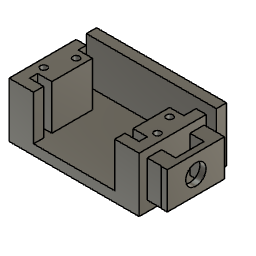
hub right down v4 (Autodesk Fusion 360 design; units mm, degrees)
Autodesk Fusion 360 part; units mm, degrees
sketch "Sketch1" plane through (0, 0, 0) normal (0, 0, 1) x (1, 0, 0) in component "casing v1"
  line L0 (-13.5, -7.7959) -> (9.5, -7.7959)
  line L1 (9.5, -7.7959) -> (9.5, -4.7959)
  line L2 (9.5, -4.7959) -> (19.5, -4.7959)
  line L3 (19.5, -4.7959) -> (19.5, 1.2041)
  line L4 (19.5, 1.2041) -> (26.5, 1.2041)
  line L5 (26.5, 1.2041) -> (26.5, 4.2041)
  line L6 (26.5, 4.2041) -> (19.5, 4.2041)
  line L7 (19.5, 4.2041) -> (19.5, 30.2041)
  line L8 (19.5, 30.2041) -> (-19.5, 30.2041)
  line L9 (-19.5, 30.2041) -> (-19.5, 4.2041)
  line L10 (-19.5, 4.2041) -> (-26.5, 4.2041)
  line L11 (-26.5, 4.2041) -> (-26.5, 1.2041)
  line L12 (-26.5, 1.2041) -> (-19.5, 1.2041)
  line L13 (-19.5, 1.2041) -> (-19.5, -4.7959)
  line L14 (-19.5, -4.7959) -> (-13.5, -4.7959)
  line L15 (-13.5, -4.7959) -> (-13.5, -7.7959)
  line L16 (-20, 0.7041) -> (-32, 0.7041)
  line L17 (-32, 0.7041) -> (-32, -4.2959)
  line L18 (-32, -4.2959) -> (-20, -4.2959)
  line L19 (-20, -4.2959) -> (-20, 0.7041)
  line L20 (-32, 0.7041) -> (-27, 0.7041)
  line L21 (-27, 0.7041) -> (-27, 38.7041)
  line L22 (-27, 38.7041) -> (-32, 38.7041)
  line L23 (-32, 38.7041) -> (-32, 0.7041)
  line L24 (-27, 38.7041) -> (27, 38.7041)
  line L25 (27, 38.7041) -> (27, 33.7041)
  line L26 (27, 33.7041) -> (-27, 33.7041)
  line L27 (-27, 33.7041) -> (-27, 38.7041)
  line L28 (20, 0.7041) -> (32, 0.7041)
  line L29 (32, 0.7041) -> (32, -4.2959)
  line L30 (32, -4.2959) -> (20, -4.2959)
  line L31 (20, -4.2959) -> (20, 0.7041)
  line L32 (32, 0.7041) -> (27, 0.7041)
  line L33 (27, 0.7041) -> (27, 38.7041)
  line L34 (27, 38.7041) -> (32, 38.7041)
  line L35 (32, 38.7041) -> (32, 0.7041)
  line L36 (27, 4.7041) -> (20, 4.7041)
  line L37 (20, 4.7041) -> (20, 22.7041)
  line L38 (20, 22.7041) -> (27, 22.7041)
  line L39 (27, 22.7041) -> (27, 4.7041)
  line L40 (-27, 4.7041) -> (-20, 4.7041)
  line L41 (-20, 4.7041) -> (-20, 24.7041)
  line L42 (-20, 24.7041) -> (-27, 24.7041)
  line L43 (-27, 24.7041) -> (-27, 4.7041)
  line L44 (-32, 38.7041) -> (32, 38.7041)
  line L45 (32, 38.7041) -> (32, -4.2959)
  line L46 (32, -4.2959) -> (-32, -4.2959)
  line L47 (-32, -4.2959) -> (-32, 38.7041)
  line L48 (-27, 33.7041) -> (-32, 33.7041)
  line L49 (-32, 33.7041) -> (-32, 28.7041)
  line L50 (-32, 28.7041) -> (-27, 28.7041)
  line L51 (-27, 28.7041) -> (-27, 33.7041)
  line L52 (27, 33.7041) -> (32, 33.7041)
  line L53 (32, 33.7041) -> (32, 28.7041)
  line L54 (32, 28.7041) -> (27, 28.7041)
  line L55 (27, 28.7041) -> (27, 33.7041)
  dimension "d34" = 0.5
  dimension "d35" = 0.5
  dimension "d36" = 5
  dimension "d37" = 12
  dimension "d38" = 0.5
  dimension "d39" = 3.5
  dimension "d40" = 5
  dimension "d41" = 0.5
  dimension "d42" = 0.5
  dimension "d43" = 12
  dimension "d44" = 5
  dimension "d45" = 0.5
  dimension "d46" = 0.5
  dimension "d47" = 0.5
  dimension "d48" = 18
  dimension "d49" = 0.5
  dimension "d50" = 0.5
  dimension "d51" = 20
  dimension "d56" = 5
  dimension "d57" = 5
  constraint horizontal L16
  constraint vertical L17
  constraint horizontal L18
  constraint vertical L19
  constraint horizontal L20
  constraint vertical L21
  constraint horizontal L22
  constraint vertical L23
  constraint horizontal L24
  constraint vertical L25
  constraint horizontal L26
  constraint vertical L27
  constraint horizontal L28
  constraint vertical L29
  constraint horizontal L30
  constraint vertical L31
  constraint horizontal L32
  constraint vertical L33
  constraint horizontal L34
  constraint vertical L35
  constraint horizontal L36
  constraint vertical L37
  constraint horizontal L38
  constraint vertical L39
  constraint coincident L33 L36.start
  constraint horizontal L40
  constraint vertical L41
  constraint horizontal L42
  constraint vertical L43
  constraint coincident L21 L40.start
  constraint horizontal L44
  constraint vertical L45
  constraint horizontal L46
  constraint vertical L47
  constraint horizontal L48
  constraint vertical L49
  constraint horizontal L50
  constraint vertical L51
  constraint coincident L47 L49.end
  constraint horizontal L52
  constraint vertical L53
  constraint horizontal L54
  constraint vertical L55
  constraint coincident L45 L53.end
  measures "d34" distance of L13 L19
  measures "d35" distance of L12 L16
  measures "d36" distance of L16.end L17.end
  measures "d37" distance of L17.end L18.end
  measures "d38" distance of L11 L21
  measures "d39" distance of L8 L26
  measures "d40" distance of L24.end L25.end
  measures "d41" distance of L4 L28
  measures "d42" distance of L3 L31
  measures "d43" distance of L29.end L30.end
  measures "d44" distance of L28.end L29.end
  measures "d45" distance of L5 L33
  measures "d46" distance of L6 L36
  measures "d47" distance of L7 L37
  measures "d48" distance of L36.end L37.end
  measures "d49" distance of L10 L40
  measures "d50" distance of L9 L41
  measures "d51" distance of L40 L42
  measures "d56" distance of L48 L50
  measures "d57" distance of L52 L54
extrude "Extrude1" add sketch "Sketch1" against normal blind 5 contours L3 L4 L5 L6 L7 L8 L9 L10 L11 L12 L13 L16 L19 L21 L26 L28 L31 L33 L36 L37 L38 L40 L41 L42 L46 L51 L55 | L3 L4 L5 L6 L7 L8 L9 L10 L11 L12 L13 L46 | L16 L17 L18 L19 L20 L46 L47 | L28 L29 L30 L31 L32 L45 L46 | L16 L20 L21 L23 L43 L47 L50 | L28 L32 L33 L35 L39 L45 L54 | L21 L23 L47 L48 L49 L50 L51 | L21 L40 L41 L42 L43 | L33 L35 L45 L52 L53 L54 L55 | L33 L36 L37 L38 L39 | L21 L22 L23 L27 L44 L47 L48 | L25 L33 L34 L35 L44 L45 L52 | L21 L24 L25 L26 L27 L33 L44 makes body 1 in component "casing v1"
extrude "Extrude2" add sketch "Sketch1" along normal blind 22 contours L16 L17 L18 L19 L20 L46 L47 | L28 L29 L30 L31 L32 L45 L46 | L16 L20 L21 L23 L43 L47 L50 | L28 L32 L33 L35 L39 L45 L54 | L21 L40 L41 L42 L43 | L33 L36 L37 L38 L39 | L21 L22 L23 L27 L44 L47 L48 | L25 L33 L34 L35 L44 L45 L52 | L21 L24 L25 L26 L27 L33 L44 bodies 1 in component "casing v1"
sketch "Sketch1 (2)" plane through (0, 0, 22) normal (0, 0, 1) x (-1, 0, 0)
  line L0 (20, 4.2959) -> (20, -0.7041)
  line L1 (20, -0.7041) -> (27, -0.7041)
  line L2 (27, -0.7041) -> (27, -4.7041)
  line L3 (27, -4.7041) -> (20, -4.7041)
  line L4 (20, -4.7041) -> (20, -24.7041)
  line L5 (20, -24.7041) -> (27, -24.7041)
  line L6 (27, -24.7041) -> (27, -28.7041)
  line L7 (27, -28.7041) -> (32, -28.7041)
  line L8 (32, -28.7041) -> (32, 4.2959)
  line L9 (32, 4.2959) -> (20, 4.2959)
  line L10 (-32, 4.2959) -> (-32, -28.7041)
  line L11 (-32, -28.7041) -> (-27, -28.7041)
  line L12 (-27, -28.7041) -> (-27, -22.7041)
  line L13 (-27, -22.7041) -> (-20, -22.7041)
  line L14 (-20, -22.7041) -> (-20, -4.7041)
  line L15 (-20, -4.7041) -> (-27, -4.7041)
  line L16 (-27, -4.7041) -> (-27, -0.7041)
  line L17 (-27, -0.7041) -> (-20, -0.7041)
  line L18 (-20, -0.7041) -> (-20, 4.2959)
  line L19 (-20, 4.2959) -> (-32, 4.2959)
  circle A0 centre (24, -20.7041) radius 1.65
  circle A1 centre (28, -8.7041) radius 1.65
  circle A2 centre (-24, -18.7041) radius 1.65
  circle A3 centre (-28, -8.7041) radius 1.65
  dimension "d1" = 3.3
  dimension "d2" = 3.3
  dimension "d3" = 3.3
  dimension "d4" = 3.3
  dimension "d5" = 4
  dimension "d6" = 4
  dimension "d7" = 4
  dimension "d8" = 4
  dimension "d9" = 4
  dimension "d10" = 4
  dimension "d11" = 4
  dimension "d12" = 4
  measures "d1" diameter of A0
  measures "d2" diameter of A1
  measures "d3" diameter of A2
  measures "d4" diameter of A3
  measures "d5" distance of L4 A0.centre
  measures "d6" distance of L5 A0.centre
  measures "d7" distance of L8 A1.centre
  measures "d8" distance of L3 A1.centre
  measures "d9" distance of L13 A2.centre
  measures "d10" distance of L14 A2.centre
  measures "d11" distance of L15 A3.centre
  measures "d12" distance of L10 A3.centre
extrude "Extrude3" cut sketch "Sketch1 (2)" against normal blind 5 contours A0 | A1 | A2 | A3 bodies 1 in component "casing v1"
sketch "Sketch1 (3)" plane through (0, 0, 0) normal (0, 0, 1) x (1, 0, 0) in component "casing v1 (1)"
  line L0 (-13.5, -7.7959) -> (9.5, -7.7959)
  line L1 (9.5, -7.7959) -> (9.5, -4.7959)
  line L2 (9.5, -4.7959) -> (19.5, -4.7959)
  line L3 (19.5, -4.7959) -> (19.5, 1.2041)
  line L4 (19.5, 1.2041) -> (26.5, 1.2041)
  line L5 (26.5, 1.2041) -> (26.5, 4.2041)
  line L6 (26.5, 4.2041) -> (19.5, 4.2041)
  line L7 (19.5, 4.2041) -> (19.5, 30.2041)
  line L8 (19.5, 30.2041) -> (-19.5, 30.2041)
  line L9 (-19.5, 30.2041) -> (-19.5, 4.2041)
  line L10 (-19.5, 4.2041) -> (-26.5, 4.2041)
  line L11 (-26.5, 4.2041) -> (-26.5, 1.2041)
  line L12 (-26.5, 1.2041) -> (-19.5, 1.2041)
  line L13 (-19.5, 1.2041) -> (-19.5, -4.7959)
  line L14 (-19.5, -4.7959) -> (-13.5, -4.7959)
  line L15 (-13.5, -4.7959) -> (-13.5, -7.7959)
  line L16 (-20, 0.7041) -> (-32, 0.7041)
  line L17 (-32, 0.7041) -> (-32, -4.2959)
  line L18 (-32, -4.2959) -> (-20, -4.2959)
  line L19 (-20, -4.2959) -> (-20, 0.7041)
  line L20 (-32, 0.7041) -> (-27, 0.7041)
  line L21 (-27, 0.7041) -> (-27, 38.7041)
  line L22 (-27, 38.7041) -> (-32, 38.7041)
  line L23 (-32, 38.7041) -> (-32, 0.7041)
  line L24 (-27, 38.7041) -> (27, 38.7041)
  line L25 (27, 38.7041) -> (27, 33.7041)
  line L26 (27, 33.7041) -> (-27, 33.7041)
  line L27 (-27, 33.7041) -> (-27, 38.7041)
  line L28 (20, 0.7041) -> (32, 0.7041)
  line L29 (32, 0.7041) -> (32, -4.2959)
  line L30 (32, -4.2959) -> (20, -4.2959)
  line L31 (20, -4.2959) -> (20, 0.7041)
  line L32 (32, 0.7041) -> (27, 0.7041)
  line L33 (27, 0.7041) -> (27, 38.7041)
  line L34 (27, 38.7041) -> (32, 38.7041)
  line L35 (32, 38.7041) -> (32, 0.7041)
  line L36 (27, 4.7041) -> (20, 4.7041)
  line L37 (20, 4.7041) -> (20, 22.7041)
  line L38 (20, 22.7041) -> (27, 22.7041)
  line L39 (27, 22.7041) -> (27, 4.7041)
  line L40 (-27, 4.7041) -> (-20, 4.7041)
  line L41 (-20, 4.7041) -> (-20, 24.7041)
  line L42 (-20, 24.7041) -> (-27, 24.7041)
  line L43 (-27, 24.7041) -> (-27, 4.7041)
  line L44 (-32, 38.7041) -> (32, 38.7041)
  line L45 (32, 38.7041) -> (32, -4.2959)
  line L46 (32, -4.2959) -> (-32, -4.2959)
  line L47 (-32, -4.2959) -> (-32, 38.7041)
  line L48 (-27, 33.7041) -> (-32, 33.7041)
  line L49 (-32, 33.7041) -> (-32, 28.7041)
  line L50 (-32, 28.7041) -> (-27, 28.7041)
  line L51 (-27, 28.7041) -> (-27, 33.7041)
  line L52 (27, 33.7041) -> (32, 33.7041)
  line L53 (32, 33.7041) -> (32, 28.7041)
  line L54 (32, 28.7041) -> (27, 28.7041)
  line L55 (27, 28.7041) -> (27, 33.7041)
  dimension "d34_1" = 0.5
  dimension "d35_1" = 0.5
  dimension "d36_1" = 5
  dimension "d37_1" = 12
  dimension "d38_1" = 0.5
  dimension "d39_1" = 3.5
  dimension "d40_1" = 5
  dimension "d41_1" = 0.5
  dimension "d42_1" = 0.5
  dimension "d43_1" = 12
  dimension "d44_1" = 5
  dimension "d45_1" = 0.5
  dimension "d46_1" = 0.5
  dimension "d47_1" = 0.5
  dimension "d48_1" = 18
  dimension "d49_1" = 0.5
  dimension "d50_1" = 0.5
  dimension "d51_1" = 20
  dimension "d56_1" = 5
  dimension "d57_1" = 5
  constraint horizontal L16
  constraint vertical L17
  constraint horizontal L18
  constraint vertical L19
  constraint horizontal L20
  constraint vertical L21
  constraint horizontal L22
  constraint vertical L23
  constraint horizontal L24
  constraint vertical L25
  constraint horizontal L26
  constraint vertical L27
  constraint horizontal L28
  constraint vertical L29
  constraint horizontal L30
  constraint vertical L31
  constraint horizontal L32
  constraint vertical L33
  constraint horizontal L34
  constraint vertical L35
  constraint horizontal L36
  constraint vertical L37
  constraint horizontal L38
  constraint vertical L39
  constraint coincident L33 L36.start
  constraint horizontal L40
  constraint vertical L41
  constraint horizontal L42
  constraint vertical L43
  constraint coincident L21 L40.start
  constraint horizontal L44
  constraint vertical L45
  constraint horizontal L46
  constraint vertical L47
  constraint horizontal L48
  constraint vertical L49
  constraint horizontal L50
  constraint vertical L51
  constraint coincident L47 L49.end
  constraint horizontal L52
  constraint vertical L53
  constraint horizontal L54
  constraint vertical L55
  constraint coincident L45 L53.end
  measures "d34_1" distance of L13 L19
  measures "d35_1" distance of L12 L16
  measures "d36_1" distance of L16.end L17.end
  measures "d37_1" distance of L17.end L18.end
  measures "d38_1" distance of L11 L21
  measures "d39_1" distance of L8 L26
  measures "d40_1" distance of L24.end L25.end
  measures "d41_1" distance of L4 L28
  measures "d42_1" distance of L3 L31
  measures "d43_1" distance of L29.end L30.end
  measures "d44_1" distance of L28.end L29.end
  measures "d45_1" distance of L5 L33
  measures "d46_1" distance of L6 L36
  measures "d47_1" distance of L7 L37
  measures "d48_1" distance of L36.end L37.end
  measures "d49_1" distance of L10 L40
  measures "d50_1" distance of L9 L41
  measures "d51_1" distance of L40 L42
  measures "d56_1" distance of L48 L50
  measures "d57_1" distance of L52 L54
extrude "Extrude1'" add sketch "Sketch1 (3)" against normal blind 5 separate body contours L3 L4 L5 L6 L7 L8 L9 L10 L11 L12 L13 L16 L19 L21 L26 L28 L31 L33 L36 L37 L38 L40 L41 L42 L46 L51 L55 | L3 L4 L5 L6 L7 L8 L9 L10 L11 L12 L13 L46 | L16 L17 L18 L19 L20 L46 L47 | L28 L29 L30 L31 L32 L45 L46 | L16 L20 L21 L23 L43 L47 L50 | L28 L32 L33 L35 L39 L45 L54 | L21 L23 L47 L48 L49 L50 L51 | L21 L40 L41 L42 L43 | L33 L35 L45 L52 L53 L54 L55 | L33 L36 L37 L38 L39 | L21 L22 L23 L27 L44 L47 L48 | L25 L33 L34 L35 L44 L45 L52 | L21 L24 L25 L26 L27 L33 L44 makes body 2 in component "casing v1 (1)"
extrude "Extrude2'" add sketch "Sketch1 (3)" along normal blind 22 contours L16 L17 L18 L19 L20 L46 L47 | L28 L29 L30 L31 L32 L45 L46 | L16 L20 L21 L23 L43 L47 L50 | L28 L32 L33 L35 L39 L45 L54 | L21 L40 L41 L42 L43 | L33 L36 L37 L38 L39 | L21 L22 L23 L27 L44 L47 L48 | L25 L33 L34 L35 L44 L45 L52 | L21 L24 L25 L26 L27 L33 L44 bodies 2 in component "casing v1 (1)"
sketch "Sketch2" plane through (0, 0, 41.3886) normal (0, 0, -1) x (1, 0, 0)
  line L0 (-31.9538, 4.2959) -> (-31.9538, -28.7041)
  line L1 (-31.9538, -28.7041) -> (-26.9538, -28.7041)
  line L2 (-26.9538, -28.7041) -> (-26.9538, -22.7041)
  line L3 (-26.9538, -22.7041) -> (-19.9538, -22.7041)
  line L4 (-19.9538, -22.7041) -> (-19.9538, -4.7041)
  line L5 (-19.9538, -4.7041) -> (-26.9538, -4.7041)
  line L6 (-26.9538, -4.7041) -> (-26.9538, -0.7041)
  line L7 (-26.9538, -0.7041) -> (-19.9538, -0.7041)
  line L8 (-19.9538, -0.7041) -> (-19.9538, 4.2959)
  line L9 (-19.9538, 4.2959) -> (-31.9538, 4.2959)
  line L10 (20.0462, 4.2959) -> (20.0462, -0.7041)
  line L11 (20.0462, -0.7041) -> (27.0462, -0.7041)
  line L12 (27.0462, -0.7041) -> (27.0462, -4.7041)
  line L13 (27.0462, -4.7041) -> (20.0462, -4.7041)
  line L14 (20.0462, -4.7041) -> (20.0462, -24.7041)
  line L15 (20.0462, -24.7041) -> (27.0462, -24.7041)
  line L16 (27.0462, -24.7041) -> (27.0462, -28.7041)
  line L17 (27.0462, -28.7041) -> (32.0462, -28.7041)
  line L18 (32.0462, -28.7041) -> (32.0462, 4.2959)
  line L19 (32.0462, 4.2959) -> (20.0462, 4.2959)
  circle A0 centre (-27.9538, -8.7041) radius 1.5
  circle A1 centre (-23.9538, -18.7041) radius 1.5
  circle A2 centre (24.0462, -20.7041) radius 1.5
  circle A3 centre (28.0462, -8.7041) radius 1.5
  dimension "d15" = 3
  dimension "d16" = 3
  dimension "d17" = 3
  dimension "d18" = 3
  dimension "d19" = 4
  dimension "d20" = 4
  dimension "d21" = 4
  dimension "d22" = 4
  dimension "d23" = 4
  dimension "d24" = 4
  dimension "d25" = 4
  dimension "d26" = 4
  measures "d15" diameter of A0
  measures "d16" diameter of A1
  measures "d17" diameter of A2
  measures "d18" diameter of A3
  measures "d19" distance of L3 A1.centre
  measures "d20" distance of L4 A1.centre
  measures "d21" distance of L0 A0.centre
  measures "d22" distance of L5 A0.centre
  measures "d23" distance of L13 A3.centre
  measures "d24" distance of L18 A3.centre
  measures "d25" distance of L14 A2.centre
  measures "d26" vertical distance of L15.end A2.centre
extrude "Extrude3'" add sketch "Sketch2" along normal blind 4.5 contours A0 | A1 | A2 | A3 sketch seen with x (-1, 0, 0) y (0, 1, 0) z (0, 0, -1) at (0.0462, 0, 63.3886) bodies 2 in component "casing v1 (1)"
sketch "Sketch3" plane through (0, 0, 0) normal (0, 0, 1) x (1, 0, 0)
  circle A0 centre (24, 18.7041) radius 1.65
  circle A1 centre (28, 8.7041) radius 1.65
  line L0 (32, -4.2959) -> (32, 28.7041)
  line L1 (32, 28.7041) -> (27, 28.7041)
  line L2 (27, 28.7041) -> (27, 22.7041)
  line L3 (27, 22.7041) -> (20, 22.7041)
  line L4 (20, 22.7041) -> (20, 4.7041)
  line L5 (20, 4.7041) -> (27, 4.7041)
  line L6 (27, 4.7041) -> (27, 0.7041)
  line L7 (27, 0.7041) -> (20, 0.7041)
  line L8 (20, 0.7041) -> (20, -4.2959)
  line L9 (20, -4.2959) -> (32, -4.2959)
  line L10 (32, 27.7041) -> (39, 27.7041)
  line L11 (39, 27.7041) -> (39, -0.2959)
  line L12 (39, -0.2959) -> (32, -0.2959)
  line L13 (32, -0.2959) -> (32, 27.7041)
  line L14 (32, 20.7041) -> (39, 20.7041)
  line L15 (39, 20.7041) -> (39, 6.7041)
  line L16 (39, 6.7041) -> (32, 6.7041)
  line L17 (32, 6.7041) -> (32, 20.7041)
  line L18 (39, 27.7041) -> (42, 27.7041)
  line L19 (42, 27.7041) -> (42, -0.4562)
  line L20 (42, -0.4562) -> (39, -0.4562)
  line L21 (39, -0.4562) -> (39, 27.7041)
  dimension "d29" = 28
  dimension "d30" = 14
  dimension "d31" = 7
  dimension "d32" = 4
  dimension "d33" = 3
  constraint horizontal L10
  constraint vertical L11
  constraint horizontal L12
  constraint vertical L13
  constraint coincident L0 L10.start
  constraint horizontal L14
  constraint vertical L15
  constraint horizontal L16
  constraint vertical L17
  constraint coincident L11 L15.end
  constraint coincident L13 L14.start
  constraint midpoint L11 L15
  constraint horizontal L18
  constraint vertical L19
  constraint horizontal L20
  constraint vertical L21
  measures "d29" distance of L10.end L11.end
  measures "d30" distance of L14 L16
  measures "d31" distance of L10.start L10.end
  measures "d32" distance of L9 L12
  measures "d33" distance of L19 L21
extrude "Extrude4" add sketch "Sketch3" along normal blind 18 separate body contours L0 L11 L12 L13 L16 L21 | L11 L15 L18 L19 L20 L21 | L0 L10 L11 L13 L14 L21 makes body 3 in component "casing v1"
sketch "Sketch4" plane through (42, 0, 0) normal (1, 0, 0) x (0, 1, 0)
  line L0 (-0.4562, 0) -> (27.7041, 0)
  line L1 (27.7041, 0) -> (27.7041, 18)
  line L2 (27.7041, 18) -> (-0.4562, 18)
  line L3 (-0.4562, 18) -> (-0.4562, 0)
  circle A0 centre (13.624, 9) radius 5
  line L4 (13.624, 18) -> (13.624, 0)
  line L5 (-0.4562, 9) -> (27.7041, 9)
  dimension "d60" = 10
  constraint midpoint L2 L4.start
  constraint midpoint L0 L4.end
  constraint midpoint L3 L5.start
  constraint midpoint L1 L5.end
  constraint coincident A0.centre L4
  constraint coincident A0.centre L5
  measures "d60" diameter of A0
extrude "Extrude5" cut sketch "Sketch4" against normal blind 3 contours A0 L4 L5 | A0 L4 L5 | A0 L4 L5 | A0 L4 L5 bodies 1 3 in component "casing v1"
copy_body "Body->Comp1" bodies 3 removing the originals makes body 4 in component "Component"
component "casing v1" placed x (1, 0, 0) y (0, 1, 0) z (0, 0, 1) at (0, 0, 0)
component "Component" placed x (1, 0, 0) y (0, 1, 0) z (0, 0, 1) at (0, 0, 0) in component "casing v1"
